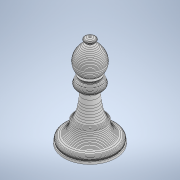
# Autodesk Inventor part: Bishop
Saved by Autodesk Inventor 2022 (Build 260153000, 153)
## iProperties
Created: 2022-05-17
Part Number: Bishop
Material: Generic
Document SubType Name: Modeling
Designer: Nick
Density: 1 g/cm^3
Appearance: Default
Author: Nick
Autodesk Inventor part; units mm, degrees
ref_plane "YZ Plane" through (0, 0, 0) normal (1, 0, 0) x (0, 1, 0)
ref_plane "XZ Plane" through (0, 0, 0) normal (0, 1, 0) x (-1, 0, 0)
ref_plane "XY Plane" through (0, 0, 0) normal (0, 0, 1) x (1, 0, 0)
sketch "Sketch1" plane through (0, 0, 0) normal (0, 0, 1) x (1, 0, 0)
  line L0 (21.5053, 8068.2338) -> (-21.5053, 8025.2062)
  line L1 (0, 8082.5594) -> (0, 8010.8806)
  line L2 (57.3476, 8018.0434) -> (28.6738, 7989.3696)
  line L3 (43.0106, 8032.3944) -> (14.3368, 8003.7206)
  line L4 (28.6738, 8046.72) -> (0, 8018.0462)
  line L5 (0, -6025.3118) -> (1896.2903, -6025.3118)
  line L6 (1896.2903, -6025.3118) -> (1896.2903, -5872.3784)
  line L7 (1896.2903, -5872.3784) -> (1835.1195, -5872.3784)
  line L8 (1835.1195, -5872.3784) -> (1816.3024, -5869.6902)
  line L9 (1816.3024, -5869.6902) -> (1805.0121, -5862.3426)
  line L10 (1805.0121, -5862.3426) -> (1800.1734, -5851.4107)
  line L11 (1800.1734, -5851.4107) -> (1800.711, -5837.9699)
  line L12 (1800.711, -5837.9699) -> (1813.6142, -5807.8625)
  line L13 (1813.6142, -5807.8625) -> (1835.1195, -5780.6225)
  line L14 (1835.1195, -5780.6225) -> (1853.6977, -5753.7409)
  line L15 (1853.6977, -5753.7409) -> (1863.3153, -5720.4078)
  line L16 (1863.3153, -5720.4078) -> (1863.6143, -5682.7733)
  line L17 (1863.6143, -5682.7733) -> (1854.2356, -5642.9886)
  line L18 (1854.2356, -5642.9886) -> (1834.821, -5603.2038)
  line L19 (1834.821, -5603.2038) -> (1805.0123, -5565.5694)
  line L20 (1805.0123, -5565.5694) -> (1764.4508, -5532.2362)
  line L21 (1764.4508, -5532.2362) -> (1712.7783, -5505.3546)
  line L22 (1712.7783, -5505.3546) -> (1606.1478, -5455.7131)
  line L23 (1606.1478, -5455.7131) -> (1496.2916, -5394.9606)
  line L24 (1496.2916, -5394.9606) -> (1441.834, -5358.7377)
  line L25 (1441.834, -5358.7377) -> (1388.5859, -5317.7205)
  line L26 (1388.5859, -5317.7205) -> (1337.2195, -5271.2375)
  line L27 (1337.2195, -5271.2375) -> (1288.4068, -5218.6168)
  line L28 (1288.4068, -5218.6168) -> (1242.8201, -5159.1861)
  line L29 (1242.8201, -5159.1861) -> (1201.1311, -5092.2731)
  line L30 (1201.1311, -5092.2731) -> (1164.0121, -5017.206)
  line L31 (1164.0121, -5017.206) -> (1132.1348, -4933.3131)
  line L32 (1132.1348, -4933.3131) -> (1106.1717, -4839.9218)
  line L33 (1106.1717, -4839.9218) -> (1086.7945, -4736.3602)
  line L34 (1086.7945, -4736.3602) -> (1074.6754, -4621.9563)
  line L35 (1074.6754, -4621.9563) -> (1070.4863, -4496.0384)
  line L36 (1070.4863, -4496.0384) -> (1031.2773, -4484.2147)
  line L37 (1031.2773, -4484.2147) -> (993.9109, -4463.4556)
  line L38 (993.9109, -4463.4556) -> (958.3478, -4434.3239)
  line L39 (958.3478, -4434.3239) -> (924.5488, -4397.3829)
  line L40 (924.5488, -4397.3829) -> (892.4747, -4353.1945)
  line L41 (892.4747, -4353.1945) -> (862.0864, -4302.3224)
  line L42 (862.0864, -4302.3224) -> (806.2099, -4182.7778)
  line L43 (806.2099, -4182.7778) -> (756.6058, -4043.2505)
  line L44 (756.6058, -4043.2505) -> (712.9604, -3888.2444)
  line L45 (712.9604, -3888.2444) -> (674.9603, -3722.2613)
  line L46 (674.9603, -3722.2613) -> (642.2916, -3549.8044)
  line L47 (642.2916, -3549.8044) -> (614.6409, -3375.3763)
  line L48 (614.6409, -3375.3763) -> (591.6944, -3203.4792)
  line L49 (591.6944, -3203.4792) -> (558.6599, -2885.2909)
  line L50 (558.6599, -2885.2909) -> (540.6791, -2631.2604)
  line L51 (540.6791, -2631.2604) -> (535.243, -2477.4078)
  line L52 (535.243, -2477.4078) -> (620.5773, -2467.4616)
  line L53 (620.5773, -2467.4616) -> (661.988, -2459.2747)
  line L54 (661.988, -2459.2747) -> (702.2895, -2445.2934)
  line L55 (702.2895, -2445.2934) -> (740.8483, -2426.0825)
  line L56 (740.8483, -2426.0825) -> (777.0307, -2402.207)
  line L57 (777.0307, -2402.207) -> (810.2031, -2374.2316)
  line L58 (810.2031, -2374.2316) -> (839.7318, -2342.7212)
  line L59 (839.7318, -2342.7212) -> (864.9833, -2308.2407)
  line L60 (864.9833, -2308.2407) -> (885.3238, -2271.3548)
  line L61 (885.3238, -2271.3548) -> (900.1198, -2232.6285)
  line L62 (900.1198, -2232.6285) -> (908.7376, -2192.6265)
  line L63 (908.7376, -2192.6265) -> (910.5436, -2151.9137)
  line L64 (910.5436, -2151.9137) -> (904.904, -2111.055)
  line L65 (904.904, -2111.055) -> (891.1854, -2070.6152)
  line L66 (891.1854, -2070.6152) -> (868.754, -2031.1591)
  line L67 (868.754, -2031.1591) -> (836.9762, -1993.2516)
  line L68 (836.9762, -1993.2516) -> (795.2183, -1957.4575)
  line L69 (795.2183, -1957.4575) -> (825.8038, -1896.2865)
  line L70 (825.8038, -1896.2865) -> (767.9187, -1880.6356)
  line L71 (767.9187, -1880.6356) -> (712.5424, -1857.0995)
  line L72 (712.5424, -1857.0995) -> (665.0515, -1826.3942)
  line L73 (665.0515, -1826.3942) -> (645.9431, -1808.5777)
  line L74 (645.9431, -1808.5777) -> (630.8222, -1789.238)
  line L75 (630.8222, -1789.238) -> (620.3607, -1768.4646)
  line L76 (620.3607, -1768.4646) -> (615.2308, -1746.3471)
  line L77 (615.2308, -1746.3471) -> (616.1045, -1722.9744)
  line L78 (616.1045, -1722.9744) -> (623.6538, -1698.4345)
  line L79 (623.6538, -1698.4345) -> (638.5507, -1672.8224)
  line L80 (638.5507, -1672.8224) -> (661.4673, -1646.2245)
  line L81 (661.4673, -1646.2245) -> (693.0756, -1618.7308)
  line L82 (693.0756, -1618.7308) -> (734.0478, -1590.4307)
  line L83 (734.0478, -1590.4307) -> (642.2919, -1498.6747)
  line L84 (642.2919, -1498.6747) -> (699.9902, -1455.8726)
  line L85 (699.9902, -1455.8726) -> (756.9271, -1397.1214)
  line L86 (756.9271, -1397.1214) -> (810.907, -1323.675)
  line L87 (810.907, -1323.675) -> (859.7344, -1236.7872)
  line L88 (859.7344, -1236.7872) -> (901.2144, -1137.7138)
  line L89 (901.2144, -1137.7138) -> (933.1513, -1027.7084)
  line L90 (933.1513, -1027.7084) -> (953.3499, -908.0249)
  line L91 (953.3499, -908.0249) -> (959.6148, -779.9192)
  line L92 (959.6148, -779.9192) -> (956.8361, -713.0994)
  line L93 (956.8361, -713.0994) -> (949.7507, -644.6451)
  line L94 (949.7507, -644.6451) -> (938.0843, -574.7113)
  line L95 (938.0843, -574.7113) -> (921.5623, -503.4564)
  line L96 (921.5623, -503.4564) -> (899.9105, -431.0365)
  line L97 (899.9105, -431.0365) -> (872.8544, -357.6086)
  line L98 (872.8544, -357.6086) -> (840.1194, -283.3294)
  line L99 (840.1194, -283.3294) -> (801.4314, -208.3562)
  line L100 (801.4314, -208.3562) -> (756.5155, -132.8445)
  line L101 (756.5155, -132.8445) -> (705.0978, -56.9524)
  line L102 (705.0978, -56.9524) -> (646.9036, 19.1635)
  line L103 (646.9036, 19.1635) -> (581.6586, 95.3468)
  line L104 (581.6586, 95.3468) -> (509.0885, 171.4403)
  line L105 (509.0885, 171.4403) -> (428.9188, 247.2875)
  line L106 (428.9188, 247.2875) -> (340.8748, 322.7319)
  line L107 (340.8748, 322.7319) -> (244.6824, 397.6162)
  line L108 (244.6824, 397.6162) -> (311.11, 465.9551)
  line L109 (311.11, 465.9551) -> (363.2006, 531.4267)
  line L110 (363.2006, 531.4267) -> (379.3893, 562.1914)
  line L111 (379.3893, 562.1914) -> (386.6175, 591.1642)
  line L112 (386.6175, 591.1642) -> (383.093, 617.9856)
  line L113 (383.093, 617.9856) -> (367.0238, 642.2987)
  line L114 (367.0238, 642.2987) -> (338.7084, 665.118)
  line L115 (338.7084, 665.118) -> (301.0738, 687.2199)
  line L116 (301.0738, 687.2199) -> (206.4509, 726.407)
  line L117 (206.4509, 726.407) -> (100.3582, 754.126)
  line L118 (100.3582, 754.126) -> (48.387, 761.8908)
  line L119 (48.387, 761.8908) -> (0, 764.6391)
  line L120 (0, 764.6391) -> (0, -6025.3118)
  line L121 (0, -6025.3118) -> (0, 764.6391)
  point P0 (0, 0)
  point P1 (646.9036, 19.1635)
  constraints: 244 end point
revolve "Revolution1" add sketch "Sketch1" angle 360 about axis through (0, -6025.3118, 0) along (0, 1, 0)
body "Solid1"
